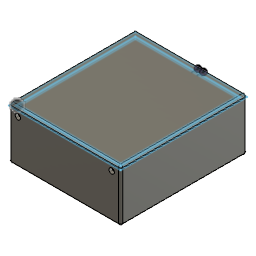
CustomBoard (Autodesk Fusion 360 design; units mm, degrees)
Autodesk Fusion 360 part; units mm, degrees
sketch "Sketch1" plane through (0, 0, 0) normal (0, 1, 0) x (1, 0, 0)
  line L0 (0, 0) -> (0, 56)
  line L1 (0, 0) -> (49, 0)
  line L2 (49, 0) -> (49, 56)
  line L3 (49, 56) -> (0, 56)
  dimension "d3" = 56
  dimension "d4" = 49
  constraint coincident L0.start L1.start
  constraint vertical L0
  constraint perpendicular L0 L1
  constraint perpendicular L1 L2
  constraint perpendicular L0 L3
  measures "d3" distance of L0.start L0.end
  measures "d4" distance of L0.start L1.end
extrude "Extrude1" add sketch "Sketch1" along normal blind 1.5 makes body 1
other "Base Mesh Feature2"
other "Modify3"
other "Modify4"
other "Modify5"
other "Modify6"
other "Scale1"
other "Modify7"
other "Base Mesh Feature3"
other "CutPasteMeshes1" in component "Boards"
other "CutPasteMeshes2" in component "Boards"
copy_body "CutPasteBodies1" bodies 1 removing the originals makes body 2 in component "Case"
copy_body "CutPasteBodies1'" bodies 2 removing the originals makes body 3 in component "Unused"
sketch "Base" plane through (0, 0, 0) normal (0, 1, 0) x (1, 0, 0) in component "Case"
  line L0 (0, 0) -> (0, 56)
  line L1 (0, 0) -> (49, 0)
  line L2 (49, 0) -> (49, 56)
  line L3 (49, 56) -> (0, 56)
  line L4 (-0.5, 56.5) -> (49.5, 56.5)
  line L5 (49.5, 56.5) -> (49.5, -0.5)
  line L6 (49.5, -0.5) -> (-0.5, -0.5)
  line L7 (-0.5, -0.5) -> (-0.5, 56.5)
  line L8 (-2, 58) -> (51, 58)
  line L9 (51, 58) -> (51, -2)
  line L10 (51, -2) -> (-2, -2)
  line L11 (-2, -2) -> (-2, 58)
  circle A0 centre (46.46, 2.54) radius 2.5
  circle A1 centre (2.54, 2.54) radius 2.5
  circle A2 centre (46.46, 53.46) radius 2.5
  circle A3 centre (2.54, 53.46) radius 2.5
  dimension "d10" = 56
  dimension "d11" = 49
  dimension "d12" = 56
  dimension "d13" = 0.5
  dimension "d14" = 0.5
  dimension "d15" = 0.5
  dimension "d16" = 0.5
  dimension "d17" = 1.5
  dimension "d18" = 1.5
  dimension "d19" = 1.5
  dimension "d20" = 1.5
  dimension "d28" = 5
  dimension "d29" = 2.54
  dimension "d30" = 2.54
  dimension "d31" = 5
  dimension "d32" = 2.54
  dimension "d33" = 2.54
  dimension "d34" = 5
  dimension "d35" = 5
  dimension "d36" = 2.54
  dimension "d37" = 2.54
  dimension "d38" = 2.54
  dimension "d39" = 2.54
  constraint coincident L0.start L1.start
  constraint vertical L0
  constraint perpendicular L0 L1
  constraint perpendicular L1 L2
  constraint horizontal L4
  constraint vertical L5
  constraint horizontal L6
  constraint vertical L7
  constraint horizontal L8
  constraint vertical L9
  constraint horizontal L10
  constraint vertical L11
  measures "d10" distance of L0.start L0.end
  measures "d11" distance of L0.start L1.end
  measures "d12" distance of L1.end L2.end
  measures "d13" distance of L3 L4
  measures "d14" distance of L2 L5
  measures "d15" distance of L0 L7
  measures "d16" distance of L1 L6
  measures "d17" distance of L5 L9
  measures "d18" distance of L4 L8
  measures "d19" distance of L7 L11
  measures "d20" distance of L6 L10
  measures "d28" diameter of A0
  measures "d29" distance of L1 A0.centre
  measures "d30" distance of L2 A0.centre
  measures "d31" diameter of A1
  measures "d32" distance of L1 A1.centre
  measures "d33" distance of L0 A1.centre
  measures "d34" diameter of A2
  measures "d35" diameter of A3
  measures "d36" distance of L3 A2.centre
  measures "d37" distance of L2 A2.centre
  measures "d38" distance of L0 A3.centre
  measures "d39" distance of L3 A3.centre
extrude "Extrude1'" add sketch "Base" along normal blind 1.5 separate body contours L0 L1 L2 L3 | L4 L5 L6 L7 | A0 | A1 | A2 | A3 makes body 4 in component "Case"
extrude "Extrude2" add sketch "Base" along normal blind 23.5 contours L8 L9 L10 L11 bodies 4 in component "Case"
fillet "Fillet2" radius 1 8 edges at (51, 11.75, -58) (51, 0, -28) (24.5, 0, -58) (-2, 0, -28) (-2, 11.75, -58) (-2, 11.75, 2) (24.5, 0, 2) (51, 11.75, 2) on bodies 4 in component "Case"
extrude "Extrude3" add sketch "Base" along normal blind 10 contours A0 | A1 | A2 | A3 bodies 4 in component "Case"
other "Modify1" in component "Boards"
ref_plane "WorkPlane1" through (0, 10, 0) normal (0, 1, 0) x (1, 0, 0) in component "Case"
sketch "ScrewHoles" plane through (0, 10, 0) normal (0, 1, 0) x (1, 0, 0) in component "Case"
  line L0 (49.5, -0.5) -> (-0.5, -0.5)
  line L1 (-0.5, 56.5) -> (49.5, 56.5)
  circle A0 centre (46.46, 53.46) radius 2.5
  line L2 (51, -2) -> (-2, -2)
  circle A1 centre (2.54, 53.46) radius 2.5
  circle A2 centre (2.54, 2.54) radius 2.5
  line L3 (49.5, 56.5) -> (49.5, -0.5)
  line L4 (49, 56) -> (0, 56)
  line L5 (49, 0) -> (49, 56)
  line L6 (0, 0) -> (49, 0)
  line L7 (-2, 58) -> (51, 58)
  line L8 (-0.5, -0.5) -> (-0.5, 56.5)
  line L9 (0, 0) -> (0, 56)
  circle A3 centre (46.46, 2.54) radius 2.5
  line L10 (-2, -2) -> (-2, 58)
  line L11 (51, 58) -> (51, -2)
  dimension "d98" = 56
  dimension "d99" = 49
  dimension "d100" = 56
  dimension "d101" = 0.5
  dimension "d102" = 0.5
  dimension "d103" = 0.5
  dimension "d104" = 0.5
  dimension "d105" = 1.5
  dimension "d106" = 1.5
  dimension "d107" = 1.5
  dimension "d108" = 1.5
  dimension "d109" = 5
  dimension "d110" = 2.54
  dimension "d111" = 2.54
  dimension "d112" = 5
  dimension "d113" = 2.54
  dimension "d114" = 2.54
  dimension "d115" = 5
  dimension "d116" = 5
  dimension "d117" = 2.54
  dimension "d118" = 2.54
  dimension "d119" = 2.54
  dimension "d120" = 2.54
  constraint coincident L6.start L9.start
  constraint vertical L9
  constraint perpendicular L6 L9
  constraint perpendicular L5 L6
  constraint horizontal L1
  constraint vertical L3
  constraint horizontal L0
  constraint vertical L8
  constraint horizontal L7
  constraint vertical L11
  constraint horizontal L2
  constraint vertical L10
  measures "d98" distance of L6.start L4.end
  measures "d99" distance of L5.start L6.start
  measures "d100" distance of L4.start L5.start
  measures "d101" distance of L1 L4
  measures "d102" distance of L3 L5
  measures "d103" distance of L8 L9
  measures "d104" distance of L0 L6
  measures "d105" distance of L3 L11
  measures "d106" distance of L1 L7
  measures "d107" distance of L8 L10
  measures "d108" distance of L0 L2
  measures "d109" diameter of A3
  measures "d110" distance of A3.centre L6
  measures "d111" distance of A3.centre L5
  measures "d112" diameter of A2
  measures "d113" distance of A2.centre L6
  measures "d114" distance of A2.centre L9
  measures "d115" diameter of A0
  measures "d116" diameter of A1
  measures "d117" distance of A0.centre L4
  measures "d118" distance of A0.centre L5
  measures "d119" distance of A1.centre L9
  measures "d120" distance of A1.centre L4
hole "Hole1" at (2.54, 10, -53.46) at (46.46, 10, -53.46) at (46.46, 10, -2.54) at (2.54, 10, -2.54) direction (0, -1, 0) diameter 2.076 depth 8 tip angle 180 bodies 4 in component "Case"
thread "Thread1" "ISO Metric profile 2.5 M2.5x0.45 6H" major diameter 2.58 minor diameter 2.0755 pitch 0.45 angle 60 resizes the face on face at (1.5023, 7.3333, -53.4859) on face at (2.6434, 7.3333, -1.5072) on face at (45.9188, 7.3333, -3.4257) on face at (45.4223, 7.3333, -53.4859) on bodies 4 in component "Case"
sketch "Ports" plane through (0, 0, -58) normal (0, 0, -1) x (-1, 0, 0) in component "Case"
  line L0 (1, 23.5) -> (-50, 23.5)
  line L1 (-24.0164, 3.5601) -> (-14.645, 3.5601)
  line L2 (-14.645, 3.5601) -> (-14.645, 7.9694)
  line L3 (-14.645, 7.9694) -> (-24.0164, 7.9694)
  line L4 (-24.0164, 7.9694) -> (-24.0164, 3.5601)
  line L5 (-39.545, 12.2897) -> (-18.4542, 12.2897)
  line L6 (-18.4542, 12.2897) -> (-18.4542, 20.6219)
  line L7 (-18.4542, 20.6219) -> (-39.545, 20.6219)
  line L8 (-39.545, 20.6219) -> (-39.545, 12.2897)
  line L9 (-30.2927, 20.6219) -> (-27.7065, 20.6219)
  line L10 (-30.2927, 20.6219) -> (-30.2927, 23.5)
  line L11 (-27.7065, 20.6219) -> (-27.7065, 23.5)
  line L12 (-50, 23.5) -> (-50, 1)
  line L13 (-50, 1) -> (1, 1)
  line L14 (1, 1) -> (1, 23.5)
  point P0 (-28.9996, 20.6219)
  constraint horizontal L1
  constraint vertical L2
  constraint horizontal L3
  constraint vertical L4
  constraint horizontal L5
  constraint vertical L6
  constraint horizontal L7
  constraint vertical L8
  constraint midpoint L7 P0
  constraint horizontal L9
  constraint midpoint P0 L9
  constraint coincident L0 L10.end
  constraint perpendicular L0 L10
  constraint coincident L0 L11.end
  constraint perpendicular L0 L11
extrude "Extrude4" cut sketch "Ports" against normal blind 1.5 contours L0 L7 L9 L10 L11 | L5 L6 L7 L8 L9 | L1 L2 L3 L4 bodies 4 in component "Case"
fillet "Fillet4" radius 0.5 8 edges at (18.4542, 12.2897, -57.25) (39.545, 12.2897, -57.25) (39.545, 20.6219, -57.25) (18.4542, 20.6219, -57.25) (14.645, 7.9694, -57.25) (24.0164, 7.9694, -57.25) (24.0164, 3.5601, -57.25) (14.645, 3.5601, -57.25) on bodies 4 in component "Case"
ref_plane "WorkPlane2" through (0, 23.5, 0) normal (0, 1, 0) x (1, 0, 0) in component "Case"
sketch "LidBorder" plane through (0, 23.5, 0) normal (0, 1, 0) x (1, 0, 0) in component "Case"
  line L0 (-2, 58) -> (51, 58)
  line L1 (-2, -2) -> (-2, 58)
  line L2 (49, 56) -> (0, 56)
  line L3 (-0.5, -0.5) -> (-0.5, 56.5)
  line L4 (49.5, 56.5) -> (49.5, -0.5)
  line L5 (51, -2) -> (-2, -2)
  line L6 (0, 0) -> (49, 0)
  line L7 (0, 0) -> (0, 56)
  line L8 (-0.5, 56.5) -> (49.5, 56.5)
  line L9 (51, 58) -> (51, -2)
  line L10 (49, 0) -> (49, 56)
  line L11 (49.5, -0.5) -> (-0.5, -0.5)
  line L12 (27.7065, 58) -> (27.7065, 56.5)
  line L13 (30.2927, 58) -> (30.2927, 56.5)
  line L14 (49.25, -0.25) -> (-0.25, -0.25)
  line L15 (-0.25, -0.25) -> (-0.25, 56.25)
  line L16 (-0.25, 56.25) -> (49.25, 56.25)
  line L17 (49.25, 56.25) -> (49.25, -0.25)
  line L18 (48.25, 55.25) -> (0.75, 55.25)
  line L19 (0.75, 55.25) -> (0.75, 0.75)
  line L20 (0.75, 0.75) -> (48.25, 0.75)
  line L21 (48.25, 0.75) -> (48.25, 55.25)
  line L22 (30.2927, 56.5) -> (30.2927, 55.25)
  line L23 (27.7065, 56.5) -> (27.7065, 55.25)
  point P0 (27.7065, 58)
  point P1 (30.2927, 58)
  dimension "d128" = 56
  dimension "d129" = 49
  dimension "d130" = 56
  dimension "d131" = 0.5
  dimension "d132" = 0.5
  dimension "d133" = 0.5
  dimension "d134" = 0.5
  dimension "d135" = 1.5
  dimension "d136" = 1.5
  dimension "d137" = 1.5
  dimension "d138" = 1.5
  dimension "d155" = 0.25
  dimension "d156" = 0.25
  dimension "d157" = 0.25
  dimension "d158" = 0.25
  dimension "d160" = 1
  dimension "d161" = 1
  dimension "d162" = 1
  dimension "d163" = 1
  constraint coincident L6.start L7.start
  constraint vertical L7
  constraint perpendicular L6 L7
  constraint perpendicular L6 L10
  constraint horizontal L8
  constraint vertical L4
  constraint horizontal L11
  constraint vertical L3
  constraint horizontal L0
  constraint vertical L9
  constraint horizontal L5
  constraint vertical L1
  constraint coincident P0 L12.start
  constraint coincident L8 L12.end
  constraint perpendicular L8 L12
  constraint coincident P1 L13.start
  constraint coincident L8 L13.end
  constraint perpendicular L8 L13
  constraint horizontal L14
  constraint vertical L15
  constraint horizontal L16
  constraint vertical L17
  constraint horizontal L18
  constraint vertical L19
  constraint horizontal L20
  constraint vertical L21
  constraint coincident L18 L22.end
  constraint perpendicular L18 L22
  constraint coincident L18 L23.end
  constraint perpendicular L18 L23
  measures "d128" distance of L6.start L2.end
  measures "d129" distance of L6.end L6.start
  measures "d130" distance of L2.start L6.end
  measures "d131" distance of L2 L8
  measures "d132" distance of L4 L10
  measures "d133" distance of L3 L7
  measures "d134" distance of L6 L11
  measures "d135" distance of L4 L9
  measures "d136" distance of L0 L8
  measures "d137" distance of L1 L3
  measures "d138" distance of L5 L11
  measures "d155" distance of L3 L15
  measures "d156" distance of L8 L16
  measures "d157" distance of L4 L17
  measures "d158" distance of L11 L14
  measures "d160" distance of L14 L20
  measures "d161" distance of L15 L19
  measures "d162" distance of L17 L21
  measures "d163" distance of L16 L18
extrude "Extrude5" add sketch "LidBorder" along normal blind 1.5 separate body makes body 5 in component "Case"
fillet "Fillet3" radius 1 8 edges at (24.5, 25, 2) (-2, 25, -28) (24.5, 25, -58) (51, 25, -28) (51, 24.25, 2) (-2, 24.25, 2) (-2, 24.25, -58) (51, 24.25, -58) on bodies 5 in component "Case"
extrude "Extrude6" add sketch "LidBorder" against normal blind 1 contours L2 L6 L7 L10 L14 L15 L16 L17 L22 L23 | L2 L16 L22 L23 | L2 L6 L7 L10 L18 L19 L20 L21 L22 L23 | L2 L18 L22 L23 bodies 5 in component "Case"
sketch "ScrewTabsFront" plane through (0, 0, -56.25) normal (0, 0, -1) x (-1, 0, 0) in component "Case"
  line L0 (-49.25, 23.5) -> (-49.25, 22.5)
  line L1 (-49.25, 22.5) -> (0.25, 22.5)
  line L2 (0.25, 22.5) -> (0.25, 23.5)
  line L3 (0.25, 23.5) -> (-49.25, 23.5)
  line L4 (-49.25, 23.5) -> (-44.25, 23.5)
  line L5 (-44.25, 23.5) -> (-44.25, 18.5)
  line L6 (-44.25, 18.5) -> (-49.25, 18.5)
  line L7 (-49.25, 18.5) -> (-49.25, 23.5)
  line L8 (0.25, 23.5) -> (-4.75, 23.5)
  line L9 (-4.75, 23.5) -> (-4.75, 18.5)
  line L10 (-4.75, 18.5) -> (0.25, 18.5)
  line L11 (0.25, 18.5) -> (0.25, 23.5)
  line L12 (-46.75, 18.5) -> (-46.75, 23.5)
  line L13 (-2.25, 18.5) -> (-2.25, 23.5)
  point P0 (-46.75, 21)
  point P1 (-2.25, 21)
  dimension "d172" = 5
  dimension "d173" = 5
  dimension "d174" = 5
  dimension "d175" = 5
  constraint horizontal L4
  constraint vertical L5
  constraint horizontal L6
  constraint vertical L7
  constraint coincident L0.start L3.end
  constraint horizontal L8
  constraint vertical L9
  constraint horizontal L10
  constraint vertical L11
  constraint coincident L2.end L3.start
  constraint midpoint L6 L12.start
  constraint midpoint L4 L12.end
  constraint midpoint L10 L13.start
  constraint midpoint L8 L13.end
  constraint midpoint L12 P0
  constraint midpoint L13 P1
  measures "d172" distance of L0.start L4.end
  measures "d173" distance of L0.start L6.end
  measures "d174" distance of L2.end L8.end
  measures "d175" distance of L2.end L10.end
extrude "Extrude7" cut sketch "LidBorder" against normal blind 1 contours L2 L16 L22 L23 | L2 L18 L22 L23 bodies 5 in component "Case"
extrude "Extrude8" add sketch "ScrewTabsFront" against normal blind 1 contours L0 L1 L3 L4 L7 L12 | L1 L6 L7 L12 | L1 L3 L4 L5 L12 | L1 L5 L6 L12 | L1 L3 L8 L9 L13 | L1 L9 L10 L13 | L1 L2 L3 L8 L11 L13 | L1 L10 L11 L13 bodies 5 in component "Case"
sketch "ScrewTabsBack" plane through (0, 0, 0.25) normal (0, 0, 1) x (1, 0, 0) in component "Case"
  line L0 (49.25, 23.5) -> (-0.25, 23.5)
  line L1 (-0.25, 23.5) -> (-0.25, 22.5)
  line L2 (-0.25, 22.5) -> (49.25, 22.5)
  line L3 (49.25, 22.5) -> (49.25, 23.5)
  line L4 (-0.25, 23.5) -> (4.75, 23.5)
  line L5 (4.75, 23.5) -> (4.75, 18.5)
  line L6 (4.75, 18.5) -> (-0.25, 18.5)
  line L7 (-0.25, 18.5) -> (-0.25, 23.5)
  line L8 (49.25, 23.5) -> (44.25, 23.5)
  line L9 (44.25, 23.5) -> (44.25, 18.5)
  line L10 (44.25, 18.5) -> (49.25, 18.5)
  line L11 (49.25, 18.5) -> (49.25, 23.5)
  line L12 (2.25, 18.5) -> (2.25, 23.5)
  line L13 (46.75, 18.5) -> (46.75, 23.5)
  point P0 (2.25, 21)
  point P1 (46.75, 21)
  dimension "d178" = 5
  dimension "d179" = 5
  dimension "d180" = 5
  dimension "d181" = 5
  constraint horizontal L4
  constraint vertical L5
  constraint horizontal L6
  constraint vertical L7
  constraint coincident L0.end L1.start
  constraint horizontal L8
  constraint vertical L9
  constraint horizontal L10
  constraint vertical L11
  constraint coincident L0.start L3.end
  constraint midpoint L6 L12.start
  constraint midpoint L4 L12.end
  constraint midpoint L10 L13.start
  constraint midpoint L8 L13.end
  constraint midpoint L12 P0
  constraint midpoint L13 P1
  measures "d178" distance of L0.end L4.end
  measures "d179" distance of L0.end L6.end
  measures "d180" distance of L0.start L8.end
  measures "d181" distance of L0.start L10.end
extrude "Extrude9" add sketch "ScrewTabsBack" against normal blind 1 contours L0 L2 L3 L8 L11 L13 | L0 L2 L8 L9 L13 | L2 L10 L11 L13 | L2 L9 L10 L13 | L0 L2 L4 L5 L12 | L0 L1 L2 L4 L7 L12 | L2 L5 L6 L12 | L2 L6 L7 L12 bodies 5 in component "Case"
hole "Hole2" at (2.25, 21, 0.25) at (46.75, 21, 0.25) direction (0, 0, -1) diameter 2.076 depth 1 tip angle 180 bodies 5 in component "Case"
thread "Thread2" "ISO Metric profile 2.5 M2.5x0.45 6H" major diameter 2.58 minor diameter 2.0755 pitch 0.45 angle 60 resizes the face on face at (46.2088, 20.1143, -0.0833) on face at (2.3534, 19.9672, -0.4167) on bodies 5 in component "Case"
hole "Hole3" at (46.75, 21, -56.25) at (2.25, 21, -56.25) direction (0, 0, 1) diameter 2.076 depth 1 tip angle 180 bodies 5 in component "Case"
thread "Thread3" "ISO Metric profile 2.5 M2.5x0.45 6H" major diameter 2.58 minor diameter 2.0755 pitch 0.45 angle 60 resizes the face on face at (2.3534, 22.0328, -55.5833) on face at (46.2088, 21.8857, -55.9167) on bodies 5 in component "Case"
fillet "Fillet1" radius 1 8 edges at (49.25, 18.5, -55.75) (44.25, 18.5, -55.75) (4.75, 18.5, -55.75) (-0.25, 18.5, -55.75) (-0.25, 18.5, -0.25) (4.75, 18.5, -0.25) (49.25, 18.5, -0.25) (44.25, 18.5, -0.25) on bodies 5 in component "Case"
hole "Hole4" at (46.75, 21, -56.25) at (2.25, 21, -56.25) direction (0, 0, -1) diameter 2.6 depth 2 tip angle 180 bodies 4 in component "Case"
hole "Hole5" at (46.75, 21, 0.25) at (2.25, 21, 0.25) direction (0, 0, 1) diameter 2.6 depth 1.75 tip angle 180 bodies 4 in component "Case"
component "Boards" placed x (1, 0, 0) y (0, 1, 0) z (0, 0, 1) at (0, 2.4, 0)
component "Case" placed x (1, 0, 0) y (0, 1, 0) z (0, 0, 1) at (0, 0, 0)
component "Unused" placed x (1, 0, 0) y (0, 1, 0) z (0, 0, 1) at (0, 0, 0)
equation "BoardLength = 56 mm"
equation "BoardWidth = 49 mm"
equation "d3 = BoardLength"
equation "d4 = BoardWidth"
equation "Wall = 1.5 mm"
equation "d6 = Wall"
equation "SpacingBetweenBoardAndWall = 0.5 mm"
equation "d10 = BoardLength"
equation "d11 = BoardWidth"
equation "d12 = BoardLength"
equation "d13 = SpacingBetweenBoardAndWall"
equation "d14 = SpacingBetweenBoardAndWall"
equation "d15 = SpacingBetweenBoardAndWall"
equation "d16 = SpacingBetweenBoardAndWall"
equation "d17 = Wall"
equation "d18 = Wall"
equation "d19 = Wall"
equation "d20 = Wall"
equation "d21 = Wall"
equation "InnerHeight = 22 mm"
equation "d24 = Wall + InnerHeight"
equation "BoardToScrew = 2.54 mm"
equation "ScrewPillarDiameter = 5 mm"
equation "d28 = ScrewPillarDiameter"
equation "d29 = BoardToScrew"
equation "d30 = BoardToScrew"
equation "d31 = ScrewPillarDiameter"
equation "d32 = BoardToScrew"
equation "d33 = BoardToScrew"
equation "d34 = ScrewPillarDiameter"
equation "d35 = ScrewPillarDiameter"
equation "d36 = BoardToScrew"
equation "d37 = BoardToScrew"
equation "d38 = BoardToScrew"
equation "d39 = BoardToScrew"
equation "ScrewPillarHeight = 8.5 mm"
equation "d41 = ScrewPillarHeight + Wall"
equation "d97 = Wall + ScrewPillarHeight"
equation "d98 = BoardLength"
equation "d99 = BoardWidth"
equation "d100 = BoardLength"
equation "d101 = SpacingBetweenBoardAndWall"
equation "d102 = SpacingBetweenBoardAndWall"
equation "d103 = SpacingBetweenBoardAndWall"
equation "d104 = SpacingBetweenBoardAndWall"
equation "d105 = Wall"
equation "d106 = Wall"
equation "d107 = Wall"
equation "d108 = Wall"
equation "d109 = ScrewPillarDiameter"
equation "d110 = BoardToScrew"
equation "d111 = BoardToScrew"
equation "d112 = ScrewPillarDiameter"
equation "d113 = BoardToScrew"
equation "d114 = BoardToScrew"
equation "d115 = ScrewPillarDiameter"
equation "d116 = ScrewPillarDiameter"
equation "d117 = BoardToScrew"
equation "d118 = BoardToScrew"
equation "d119 = BoardToScrew"
equation "d120 = BoardToScrew"
equation "d121 = ScrewLength"
equation "ScrewLength = 8 mm"
equation "d125 = -Wall"
equation "d127 = Wall + InnerHeight"
equation "d128 = BoardLength"
equation "d129 = BoardWidth"
equation "d130 = BoardLength"
equation "d131 = SpacingBetweenBoardAndWall"
equation "d132 = SpacingBetweenBoardAndWall"
equation "d133 = SpacingBetweenBoardAndWall"
equation "d134 = SpacingBetweenBoardAndWall"
equation "d135 = Wall"
equation "d136 = Wall"
equation "d137 = Wall"
equation "d138 = Wall"
equation "d151 = Wall"
equation "LidBorderHeight = 0.5 mm"
equation "LidBorderSpacing = 0.25 mm"
equation "d155 = LidBorderSpacing"
equation "d156 = LidBorderSpacing"
equation "d157 = LidBorderSpacing"
equation "d158 = LidBorderSpacing"
equation "LidBorderThickness = 1 mm"
equation "d160 = LidBorderThickness"
equation "d161 = LidBorderThickness"
equation "d162 = LidBorderThickness"
equation "d163 = LidBorderThickness"
equation "d164 = -LidBorderThickness"
equation "LidScrewTabHeight = 5 mm"
equation "LidScrewTabWidth = 5 mm"
equation "d170 = -LidBorderThickness"
equation "d172 = LidScrewTabWidth"
equation "d173 = LidScrewTabHeight"
equation "d174 = LidScrewTabWidth"
equation "d175 = LidScrewTabHeight"
equation "d176 = -LidBorderThickness"
equation "d178 = LidScrewTabWidth"
equation "d179 = LidScrewTabHeight"
equation "d180 = LidScrewTabWidth"
equation "d181 = LidScrewTabHeight"
equation "d182 = -LidBorderThickness"
equation "d184 = LidBorderThickness"
equation "d187 = LidBorderThickness"
equation "Filet = 1 mm"
equation "d194 = Filet"
equation "d196 = Filet"
equation "d206 = Wall + SpacingBetweenBoardAndWall"
equation "d207 = ScrewPassthroughDmtr"
equation "ScrewPassthroughDmtr = 2.6 mm"
equation "d210 = Wall + LidBorderSpacing"
equation "d211 = ScrewPassthroughDmtr"
equation "d214 = Filet / 2"
named bodies: "Box", "Lid"
